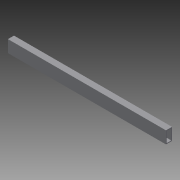
# Autodesk Inventor part: 26in box beam
Saved by Autodesk Inventor 2015 (Build 190159000, 159)
## iProperties
Created: 2015-01-11
Part Number: 26in box beam
Material: Generic
Document SubType Name: Modeling
Designer: chapale16
Density: 1 g/cm^3
Appearance: Default
Author: chapale16
Autodesk Inventor part; units mm, degrees
ref_plane "YZ Plane" through (0, 0, 0) normal (1, 0, 0) x (0, 1, 0)
ref_plane "XZ Plane" through (0, 0, 0) normal (0, 1, 0) x (-1, 0, 0)
ref_plane "XY Plane" through (0, 0, 0) normal (0, 0, 1) x (1, 0, 0)
sketch "Sketch1" plane through (0, 0, 0) normal (1, 0, 0) x (0, 1, 0)
  line L0 (5.0816, 6.2276) -> (-45.7184, 6.2276)
  line L1 (-45.7184, 6.2276) -> (-45.7184, -19.1724)
  line L2 (-45.7184, -19.1724) -> (5.0816, -19.1724)
  line L3 (5.0816, -19.1724) -> (5.0816, 6.2276)
  line L4 (1.9574, 3.1034) -> (-42.5942, 3.1034)
  line L5 (-42.5942, 3.1034) -> (-42.5942, -16.0482)
  line L6 (-42.5942, -16.0482) -> (1.9574, -16.0482)
  line L7 (1.9574, -16.0482) -> (1.9574, 3.1034)
  point P0 (0, 0)
  dimension "d0" = 50.8
  dimension "d1" = 25.4
  dimension "d2" = 3.1242
  constraints: 16 end point, 4 parallel, 2 perpendicular, 1 horizontal, 3 other
  measures "d0" distance of L2.end L1.end
  measures "d1" distance of L1.end L0.end
  measures "d2" distance between parallel lines of L3 L7
extrude "Extrusion1" add sketch "Sketch1" along normal blind 660.4
body "Solid1"
